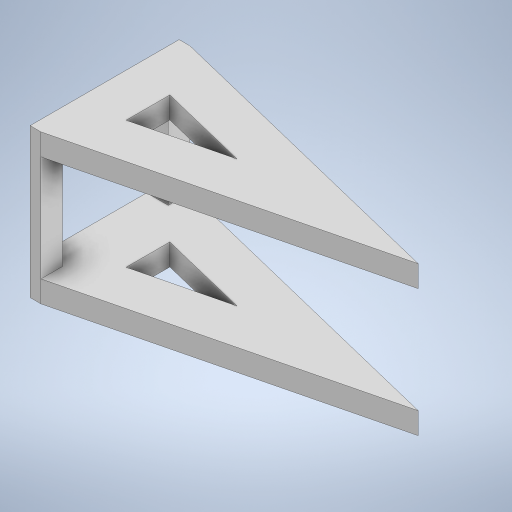
# Autodesk Inventor part: board support
Saved by Autodesk Inventor 2024 (Build 280153000, 153)
## iProperties
Created: 2024-04-17
Part Number: board support
Material: Generic
Document SubType Name: Modeling
Designer: drew
Density: 1 g/cm^3
Appearance: Default
Author: drew
Autodesk Inventor part; units mm, degrees
ref_plane "YZ Plane" through (0, 0, 0) normal (1, 0, 0) x (0, 1, 0)
ref_plane "XZ Plane" through (0, 0, 0) normal (0, 1, 0) x (-1, 0, 0)
ref_plane "XY Plane" through (0, 0, 0) normal (0, 0, 1) x (1, 0, 0)
sketch "Sketch1" plane through (0, 0, 0) normal (1, 0, 0) x (0, 1, 0)
  line L0 (-9.3345, 9.3345) -> (9.3345, 9.3345)
  line L1 (9.3345, 9.3345) -> (9.3345, -9.3345)
  line L2 (9.3345, -9.3345) -> (-9.3345, -9.3345)
  line L3 (-9.3345, -9.3345) -> (-9.3345, 9.3345)
  line L4 (-9.3345, 9.3345) -> (9.3345, -9.3345) construction
  line L5 (9.3345, 9.3345) -> (-9.3345, -9.3345) construction
  line L6 (7.747, -7.747) -> (7.747, 7.747)
  line L7 (7.747, 7.747) -> (-7.747, 7.747)
  line L8 (-7.747, 7.747) -> (-7.747, -7.747)
  line L9 (-7.747, -7.747) -> (7.747, -7.747)
  point P0 (0, 0)
  dimension "d0" = 18.669
  dimension "d1" = 1.5875
  constraints: 20 end point, 4 parallel, 3 perpendicular, 2 midpoint, 1 horizontal, 3 other
  measures "d0" distance of L1.end L2.end
  measures "d1" distance between parallel lines of L1 L6
extrude "Extrusion1" add sketch "Sketch1" along normal blind 1.5875
sketch "Sketch2" plane through (1.5875, 0, 0) normal (1, 0, 0) x (0, 0, -1)
  line L0 (9.3345, -9.3345) -> (9.3345, 9.3345) projected
  line L1 (9.3345, 9.3345) -> (-9.3345, 9.3345) projected
  line L2 (-9.3345, 9.3345) -> (-9.3345, -9.3345) projected
  line L3 (-9.3345, -9.3345) -> (9.3345, -9.3345) projected
  line L4 (7.747, 7.747) -> (7.747, -7.747) projected
  line L5 (7.747, -7.747) -> (-7.747, -7.747) projected
  line L6 (-7.747, -7.747) -> (-7.747, 7.747) projected
  line L7 (-7.747, 7.747) -> (7.747, 7.747) projected
  line L8 (-10.922, 10.922) -> (10.922, 10.922)
  line L9 (10.922, 10.922) -> (10.922, -10.922)
  line L10 (10.922, -10.922) -> (-10.922, -10.922)
  line L11 (-10.922, -10.922) -> (-10.922, 10.922)
  point P0 (0, 0)
  dimension "d4" = 1.5875
  constraints: 8 end point, 3 other
  measures "d4" distance between parallel lines of L1 L8
extrude "Extrusion2" add sketch "Sketch2" along normal blind 1.5875 contours L3 L2 L1 L0 | L8 L9 L10 L11
sketch "Sketch3" plane through (3.175, 0, 0) normal (1, 0, 0) x (0, 0, -1)
  point P0 (0, 0)
sketch "Sketch4" plane through (1.5875, 10.922, 10.922) normal (0, 1, 0) x (1, 0, 0)
  line L0 (0, 21.844) -> (0, 0) projected
  line L1 (1.5875, 0) -> (45.974, 10.922)
  line L2 (45.974, 10.922) -> (1.5875, 21.844)
  line L3 (1.5875, 21.844) -> (1.5875, 0) projected
  line L4 (6.35, 14.1327) -> (6.35, 7.7113)
  line L5 (6.35, 7.7113) -> (19.3981, 10.922)
  line L6 (19.3981, 10.922) -> (6.35, 14.1327)
  point P0 (-1.5875, 10.922)
  point P1 (1.5875, 10.922)
  dimension "d7" = 45.974
  dimension "d8" = 6.35
  constraints: 10 end point, 1 horizontal alignment, 1 midpoint, 2 other
  measures "d7" distance from line of L0 L1.end
  measures "d8" distance between parallel lines of L2 L6
extrude "Extrusion3" add sketch "Sketch4" against normal up to surface (3.175 mm away)
mirror "Mirror1" about plane through (0, 0, 0) normal (0, 1, 0) of "Extrusion3"
body "Solid1"
